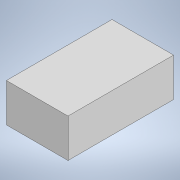
# Autodesk Inventor part: Main
Saved by Autodesk Inventor 2020 (Build 240168000, 168)
## iProperties
Created: 2020-03-14
Part Number: Main
Material: Generic
Document SubType Name: Modeling
Designer: atmat
Density: 1 g/cm^3
Appearance: Default
Author: atmat
Autodesk Inventor part; units mm, degrees
ref_plane "YZ Plane" through (0, 0, 0) normal (1, 0, 0) x (0, 1, 0)
ref_plane "XZ Plane" through (0, 0, 0) normal (0, 1, 0) x (-1, 0, 0)
ref_plane "XY Plane" through (0, 0, 0) normal (0, 0, 1) x (1, 0, 0)
sketch "Sketch1" plane through (0, 0, 0) normal (0, 1, 0) x (-1, 0, 0)
  line L0 (28, 48) -> (-28, 48)
  line L1 (-28, 48) -> (-28, -48)
  line L2 (-28, -48) -> (28, -48)
  line L3 (28, -48) -> (28, 48)
  point P0 (0, 0)
  dimension "d0" = 96
  dimension "d1" = 56
  dimension "d2" = 28
  dimension "d3" = 48
  constraints: 8 end point, 2 parallel, 1 horizontal, 1 perpendicular
  measures "d0" distance of L2.end L0.start
  measures "d1" distance of L1.end L2.end
  measures "d2" distance from line of point (0, 0) L3
  measures "d3" distance from line of point (0, 0) L2
extrude "Extrusion1" add sketch "Sketch1" along normal blind 35
body "Solid1"
